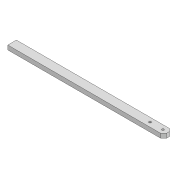
# Autodesk Inventor part: spazzola - asta
Saved by Autodesk Inventor 2022 (Build 260153000, 153)
## iProperties
Created: 2025-08-09
Part Number: spazzola - asta
Material: Generic
Document SubType Name: Modeling
Designer: sacchie
Density: 1 g/cm^3
Appearance: Default
Author: sacchie
Autodesk Inventor part; units mm, degrees
ref_plane "YZ Plane" through (0, 0, 0) normal (1, 0, 0) x (0, 1, 0)
ref_plane "XZ Plane" through (0, 0, 0) normal (0, 1, 0) x (-1, 0, 0)
ref_plane "XY Plane" through (0, 0, 0) normal (0, 0, 1) x (1, 0, 0)
sketch "Sketch1" plane through (0, 0, 0) normal (0, 0, 1) x (1, 0, 0)
  line L0 (0, 0) -> (-19, 0)
  line L1 (-19, 0) -> (-19, 0)
  line L2 (-19, 0) -> (-109, 0)
  line L3 (-109, 0) -> (-109, 3)
  line L4 (-109, 3) -> (-17, 3)
  line L5 (-17, 3) -> (-17, 3)
  line L6 (-17, 3) -> (0, 3)
  line L7 (0, 3) -> (0, 0)
  dimension "d1" = 0
  dimension "d3" = 3
  dimension "d4" = 3
  dimension "d5" = 17
  dimension "d6" = 2
  dimension "d7" = 90
  constraints: 16 end point, 6 perpendicular, 1 horizontal, 1 vertical
  measures "d1" distance of L4.end L5.end
  measures "d3" distance between parallel lines of L4 L2
  measures "d4" distance between parallel lines of L6 L0
  measures "d5" distance between parallel lines of L7 L5
  measures "d6" distance between parallel lines of L5 L1
  measures "d7" distance of L1.end L2.end
extrude "Extrusion1" add sketch "Sketch1" along normal blind 6
chamfer "Chamfer1" distance 2 angle 45 2 edges at (0, 1.5, 0) (0, 1.5, 6)
sketch "Sketch3" plane through (-109, 0, 0) normal (-1, 0, 0) x (0, 0, 1)
  line L0 (3, 0) -> (3, 4.5868) construction
  line L1 (0.8, 1.5) -> (1.5, 0)
  line L2 (1.5, 0) -> (4.5, 0)
  line L3 (4.5, 0) -> (5.2, 1.5)
  line L4 (5.2, 1.5) -> (0.8, 1.5)
  line L5 (0, 0) -> (6, 0) projected
  point P0 (0, 0)
  dimension "d20" = 1.5
  dimension "d21" = 2.2
  dimension "d22" = 4.4
  dimension "d23" = 3
  dimension "d24" = 1.5
  constraints: 10 end point, 1 collinear, 1 vertical
  measures "d20" distance from line of L0 L1.end
  measures "d21" distance from line of L1.start L0
  measures "d22" distance of L3.end L1.start
  measures "d23" distance of L2.end L1.end
  measures "d24" distance between parallel lines of L2 L4
extrude "Extrusion3" cut sketch "Sketch3" against normal blind 87
sketch "Sketch4" plane through (-109, 3, 6) normal (0, 1, 0) x (1, 0, 0)
  line L0 (109, 4) -> (109, 2) projected
  line L1 (109, 3) -> (86.5142, 3) construction
  circle A0 centre (96.5, 3) radius 0.75
  circle A1 centre (105.5, 3) radius 0.75
  point P0 (109, 6)
  dimension "d42" = 3.5
  dimension "d43" = 9
  dimension "d44" = 1.5
  dimension "d45" = 1.5
  constraints: 2 centre point, 2 end point, 2 point on line, 1 horizontal, 1 midpoint
  measures "d42" distance from line of L0 A1.centre
  measures "d43" distance of A0.centre A1.centre
  measures "d44" diameter of A0
  measures "d45" diameter of A1
extrude "Extrusion4" cut sketch "Sketch4" against normal through all
equation "\"d20\" = 0.5 * d23"
equation "\"d21\" = 0.5 * d22"
body "Solid1"
